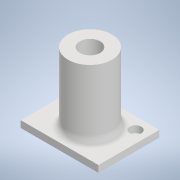
# Autodesk Inventor part: 11_Connettore_MPU
Saved by Autodesk Inventor 2020 (Build 240168000, 168)
## iProperties
Created: 2019-10-15
Part Number: 11_Connettore_MPU
Material: Generico
Document SubType Name: Modeling
Designer: socci
Density: 1 g/cm^3
Appearance: Default
Author: socci
Autodesk Inventor part; units mm, degrees
ref_plane "YZ Plane" through (0, 0, 0) normal (1, 0, 0) x (0, 1, 0)
ref_plane "XZ Plane" through (0, 0, 0) normal (0, 1, 0) x (-1, 0, 0)
ref_plane "XY Plane" through (0, 0, 0) normal (0, 0, 1) x (1, 0, 0)
sketch "Schizzo1" plane through (0, 0, 0) normal (0, 1, 0) x (-1, 0, 0)
  circle A0 centre (0, 0) radius 3
  circle A1 centre (0, 0) radius 6.5
  dimension "d0" = 6
  dimension "d1" = 13
  constraints: 2 centre point, 2 coincident
  measures "d0" diameter of A0
  measures "d1" diameter of A1
extrude "Estrusione1" add sketch "Schizzo1" along normal blind 20
sketch "Schizzo2" plane through (0, 0, 0) normal (0, -1, 0) x (1, 0, 0)
  line L0 (-11.5, -9) -> (11.5, -9)
  line L1 (11.5, -9) -> (11.5, 9)
  line L2 (11.5, 9) -> (-11.5, 9)
  line L3 (-11.5, 9) -> (-11.5, -9)
  line L4 (-11.5, -9) -> (11.5, 9) construction
  line L5 (11.5, -9) -> (-11.5, 9) construction
  point P0 (0, 0)
  point P1 (0, 0)
  point P2 (0, 0)
  dimension "d4" = 18
  dimension "d5" = 23
  constraints: 12 end point, 3 midpoint, 2 parallel, 1 coincident, 1 horizontal, 1 perpendicular
  measures "d4" distance of L2.end L0.start
  measures "d5" distance of L0.start L0.end
extrude "Estrusione2" add sketch "Schizzo2" along normal blind 2
fillet "Raccordo1" radius 2 1 edges at (6.5, 0, 0)
sketch "Schizzo3" plane through (0, -2, 0) normal (0, -1, 0) x (1, 0, 0)
  line L0 (-11.5, -9) -> (11.5, -9) projected
  line L1 (11.5, -9) -> (8, -9)
  line L2 (8, -9) -> (8, -5.5)
  line L3 (-11.5, -9) -> (11.5, -9) projected
  line L4 (-11.5, -9) -> (-8, -9)
  line L5 (-8, -9) -> (-8, -5.5)
  point P0 (0, 0)
  point P1 (2.8723, -8)
  dimension "d10" = 3.5
  dimension "d11" = 3.5
  dimension "d12" = 3.5
  dimension "d13" = 3.5
  constraints: 8 end point, 2 perpendicular, 4 other
  measures "d10" distance of L1.start L1.end
  measures "d11" distance of L1.end L2.end
  measures "d12" distance of L4.start L4.end
  measures "d13" distance of L4.end L5.end
hole "Foro1" at (8, -2, -5.5) at (-8, -2, -5.5) direction (0, 1, 0) diameter 3.4 end through all clearance for "Vite a testa esagonale" size "M3" standard "ANSI - Profilo M Metrico"
